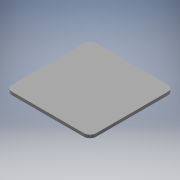
# Autodesk Inventor part: PistonFeederHeadMini
Saved by Autodesk Inventor 2016 (Build 200138000, 138)
## iProperties
Created: 2015-08-02
Part Number: PistonFeederHeadMini
Material: Stainless Steel
Document SubType Name: Modeling
Designer: myhome
Density: 8 g/cm^3
Appearance: Semi-Polished
Mass: 174.242 g
Surface Area: 121.152 cm^2
Volume: 21.7802 cm^3
Author: myhome
Autodesk Inventor part; units mm, degrees
ref_plane "YZ Plane" through (0, 0, 0) normal (1, 0, 0) x (0, 1, 0)
ref_plane "XZ Plane" through (0, 0, 0) normal (0, 1, 0) x (-1, 0, 0)
ref_plane "XY Plane" through (0, 0, 0) normal (0, 0, 1) x (1, 0, 0)
sketch "Sketch1" plane through (0, 0, 0) normal (0, 0, 1) x (1, 0, 0)
  line L0 (8, 0) -> (102, 0)
  line L1 (110, 8) -> (110, 102)
  line L2 (102, 110) -> (8, 110)
  line L3 (0, 102) -> (0, 8)
  arc A0 (2.5, 110) -> (0, 107.5) centre (2.5, 107.5) ccw
  arc A1 (110, 102) -> (102, 110) centre (102, 102) ccw
  arc A2 (8, 110) -> (0, 102) centre (8, 102) ccw
  arc A3 (0, 8) -> (8, 0) centre (8, 8) ccw
  arc A4 (102, 0) -> (110, 8) centre (102, 8) ccw
  circle A5 centre (55, 55) radius 5
  point P0 (0, 0)
  point P1 (110, 110)
  point P2 (110, 0)
  point P3 (0, 110)
  dimension "d0" = 110
  dimension "d1" = 110
  dimension "d3" = 8
  dimension "d4" = 8
  dimension "d6" = 8
  dimension "d9" = 10
  constraints: 10 point on circle, 10 point on line, 10 tangent, 8 end point, 6 centre point, 2 parallel, 1 equal radius, 1 horizontal, 1 perpendicular
  measures "d0" distance of point (110, 110) point (0, 110)
  measures "d1" distance of point (110, 0) point (110, 110)
  measures "d3" radius of A1
  measures "d4" radius of A2
  measures "d6" radius of A4
  measures "d9" diameter of A5
extrude "Extrusion1" add sketch "Sketch1" along normal blind 4 contours A3 L3 A2 L2 A1 L1 A4 L0 | A5
body "Solid1"
